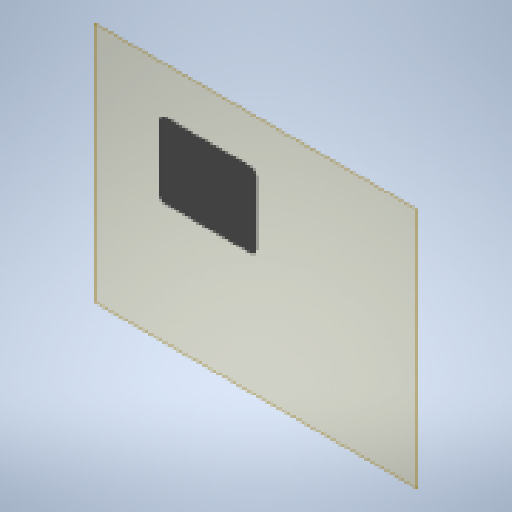
# Autodesk Inventor part: Alfombras
Saved by Autodesk Inventor 2024 (Build 280153000, 153)
## iProperties
Created: 2024-04-05
Part Number: Alfombras
Material: Genérico
Document SubType Name: Modeling
Designer: sergi
Density: 1 g/cm^3
Appearance: Valor por defecto
Author: sergi
Autodesk Inventor part; units mm, degrees
ref_plane "YZ Plane" through (0, 0, 0) normal (1, 0, 0) x (0, 1, 0)
ref_plane "XZ Plane" through (0, 0, 0) normal (0, 1, 0) x (-1, 0, 0)
ref_plane "XY Plane" through (0, 0, 0) normal (0, 0, 1) x (1, 0, 0)
ref_plane "Plano de trabajo1" through (-30.1886, 64.9106, 0) normal (0, 0, 1) x (1, 0, 0)
sketch "Boceto1" plane through (-30.1886, 64.9106, 0) normal (0, 0, 1) x (1, 0, 0)
  line L0 (30.1886, -64.9106) -> (-1369.8114, -64.9106)
  line L1 (-1369.8114, -64.9106) -> (-1369.8114, 1735.0894)
  line L2 (-1369.8114, 1735.0894) -> (30.1886, 1735.0894)
  line L3 (30.1886, 1735.0894) -> (30.1886, -64.9106)
  dimension "d0" = 1400
  dimension "d1" = 1800
  constraints: 8 end point, 2 parallel, 1 horizontal, 1 perpendicular
  measures "d0" distance of L1.end L2.end
  measures "d1" distance of L0.end L1.end
extrude "Extrusión1" add sketch "Boceto1" along normal blind 3
fillet "Empalme1" radius 100 4 edges at (0, 0, 1.5) (-1400, 0, 1.5) (-1400, 1800, 1.5) (0, 1800, 1.5)
